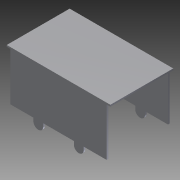
# Autodesk Inventor part: M20_ang_t_shorud1230TX-switch
Saved by Autodesk Inventor 2011 SP1 (Build 150282100, 282)
## iProperties
Created: 2013-12-24
Part Number: M20_ang_t_shorud1230TX-switch
Catalog Web Link: www.cadenas.de
Description: Angle Mount Miniature Rockers- Switch - Shroud-Series M - Miniature Toggle
Vendor: NKKSWITCHES
Document SubType Name: Modeling
Designer: PARTuser1
Manufacturer: NKKSWITCHES
Density: 1 g/cm^3
Category: PARTsolutions
Company: NKKSWITCHES
Title: M20_ang_t_shorud1230TX-switch
Author: Cadenas PARTsolutions
Comments: Series M - Miniature Toggle
PSOL_IDENT_0: {$CADENAS_DATA\23d-libs\nkkswitches\toggle\m\parts\m_ang_t_shroud.prj},260 {VTYP=3D},{NB=M20_ang_t_s
PSOL_IDENT_1: horud1230TX-switch},{LINA=M20_ang_t_shorud1230TX-switch},{NN=Angle Mount Miniature Rockers- Switch -
PSOL_IDENT_2: Shroud},{DATE=28.05.2007 07:44:41},{GEOMDATE=28.05.2007 00:00:00},{VERSION=},{LINEID=10},{LINESUBID
PSOL_IDENT_3: =-1},{WBVAR=PLS,CRCTS,FRM,TRMNLS}  {NB=M20_ang_t_shorud1230TX-switch},{LINA=M20_ang_t_shorud1230TX-s
PSOL_IDENT_4: witch},{KT=DUMMY},{PN=M20_ang_t_shorud1230TX},{SRS=M20},{PLS=1},{CRCTSALG='2','2 - ON/NONE/ON','3','
PSOL_IDENT_5: 3 - ON/OFF/ON','5','5 - ON/NONE/(ON)','8','8 - (ON)/OFF/(ON)','9','9 - ON/OFF/(ON)','4', '4 - ON/ON/
PSOL_IDENT_6: ON','6','6 - (ON)/ON/(ON)','7','7 - ON/ON/(ON)'},{CRCTS=2},{FRMALG='TX', 'TX - Narrow Frame for Smal
PSOL_IDENT_7: l Actuator', 'TZ'  , 'TZ - Wide Frame for Large Actuator'},{FRM=TX},{TRMNLSALG='30', '30 - .150\" (3
PSOL_IDENT_8: .81mm) Right Angle PC (1-3 Pole)', '32'  , '32 -  Right Angle PCB (1 Pole & 0.4VA Rating Only', '40'
PSOL_IDENT_9: , '40 - .150\" (3.81mm) Vertical PC (1-4 Pole)', '45'  , '45 - .100\" (2.54mm) Vertical PC (1-4 Po
PSOL_IDENT_10: le)'},{TRMNLS=30},{WIDTH=0.512},{HEIGHT=0.3877},{LENGTH=0.311},{A=0.15},{TRMNLNOH=1},{TRMNLOV=3},{LT
PSOL_IDENT_11: RMNL=0.031},{POS=0},{POS2=0.185},{POS3=0},{D=0},{HOLES=0.185},{WH=0.00000},{D1=0.00000},{D2=0.00000}
CNS_NN: Angle Mount Miniature Rockers- Switch - Shroud
CNS_NT: Series M - Miniature Toggle
CNS_NB: M20_ang_t_shorud1230TX-switch
CNS_NBSYN: $PN.-switch
CNS_LINA: M20_ang_t_shorud1230TX-switch
CNS_PN: M20_ang_t_shorud1230TX
CNS_SRS: M20
CNS_PLS: 1 - SPST/SPDT
CNS_CRCTSALG: '2','2 - ON/NONE/ON','3','3 - ON/OFF/ON','5','5 - ON/NONE/(ON)','8','8 - (ON)/OFF/(ON)','9','9 - ON/OFF/(ON)','4', '4 - ON/ON/ON','6','6 - (ON)/ON/(ON)','7','7 - ON/ON/(ON)'
CNS_CRCTS: 2 - ON/NONE/ON
CNS_FRMALG: 'TX', 'TX - Narrow Frame for Small Actuator', 'TZ'  , 'TZ - Wide Frame for Large Actuator'
CNS_FRM: TX - Narrow Frame for Small Actuator
CNS_TRMNLSALG: '30', '30 - .150" (3.81mm) Right Angle PC (1-3 Pole)', '32'  , '32 -  Right Angle PCB (1 Pole & 0.4VA Rating Only', '40'  , '40 - .150" (3.81mm) Vertical PC (1-4 Pole)', '45'  , '45 - .100" (2.54mm) Vertical PC (1-4 Pole)'
CNS_TRMNLS: 30 - .150" (3.81mm) Right Angle PC (1-3 Pole)
CNS_WIDTH: 0.512
CNS_HEIGHT: 0.388
CNS_LENGTH: 0.311
CNS_A: 0.150
CNS_TRMNLNOH: 1.000
CNS_TRMNLOV: 3.000
CNS_LTRMNL: 0.031
CNS_POS: 0.000
CNS_POS2: 0.185
CNS_POS3: 0.000
CNS_D: 0.000
CNS_HOLES: 0.185
CNS_WH: 0.00000
CNS_D1: 0.00000
CNS_D2: 0.00000
SUPPLIER: NKKSWITCHES
ARTICLENO: M20_ang_t_shorud1230TX-switch
BOMINFO: M20_ang_t_shorud1230TX-switch
CREATOR: CADENAS GmbH
Autodesk Inventor part; units mm, degrees
sketch "Sketch_1" plane through (0, 0, 0) normal (0, 1, 0) x (-1, 0, 0)
  line L0 (6.5024, 3.9497) -> (-6.5024, 3.9497)
  line L1 (-6.5024, 3.9497) -> (-6.5024, -3.9497)
  line L2 (-6.5024, -3.9497) -> (6.5024, -3.9497)
  line L3 (6.5024, -3.9497) -> (6.5024, 3.9497)
  constraints: 8 end point
extrude "Extrusion1" add sketch "Sketch_1" along normal blind 0.2032
sketch "Sketch_2" plane through (0, 0, -3.9497) normal (0, 0, 1) x (1, 0, 0)
  line L0 (-6.0389, -6.018) -> (-3.1581, -6.018)
  line L1 (-3.1581, -6.018) -> (-3.1581, -6.4159)
  arc A0 (-3.1581, -6.4159) -> (-1.9219, -6.4159) centre (-2.54, -6.4159) ccw
  line L2 (-1.9219, -6.4159) -> (-1.9219, -6.018)
  line L3 (-1.9219, -6.018) -> (1.9219, -6.018)
  line L4 (1.9219, -6.018) -> (1.9219, -6.4159)
  arc A1 (1.9219, -6.4159) -> (3.1581, -6.4159) centre (2.54, -6.4159) ccw
  line L5 (3.1581, -6.4159) -> (3.1581, -6.018)
  line L6 (3.1581, -6.018) -> (6.0389, -6.018)
  line L7 (6.0389, -6.018) -> (6.0389, 0)
  line L8 (6.0389, 0) -> (-6.0389, 0)
  line L9 (-6.0389, 0) -> (-6.0389, -6.018)
  constraints: 20 end point, 4 point on circle, 2 centre point
extrude "Extrusion2" add sketch "Sketch_2" along normal blind 0.2032
sketch "Sketch_3" plane through (0, 0, 3.9497) normal (0, 0, 1) x (1, 0, 0)
  line L0 (-6.0389, -6.018) -> (-3.1581, -6.018)
  line L1 (-3.1581, -6.018) -> (-3.1581, -6.4159)
  arc A0 (-3.1581, -6.4159) -> (-1.9219, -6.4159) centre (-2.54, -6.4159) ccw
  line L2 (-1.9219, -6.4159) -> (-1.9219, -6.018)
  line L3 (-1.9219, -6.018) -> (1.9219, -6.018)
  line L4 (1.9219, -6.018) -> (1.9219, -6.4159)
  arc A1 (1.9219, -6.4159) -> (3.1581, -6.4159) centre (2.54, -6.4159) ccw
  line L5 (3.1581, -6.4159) -> (3.1581, -6.018)
  line L6 (3.1581, -6.018) -> (6.0389, -6.018)
  line L7 (6.0389, -6.018) -> (6.0389, 0)
  line L8 (6.0389, 0) -> (-6.0389, 0)
  line L9 (-6.0389, 0) -> (-6.0389, -6.018)
  constraints: 20 end point, 4 point on circle, 2 centre point
extrude "Extrusion3" add sketch "Sketch_3" against normal blind 0.2032
ref_plane "shroud_to_body_XY" through (0, 0, 0) normal (0, 1, 0) x (1, 0, 0)
ref_plane "shroud_to_body_YZ" through (0, 0, 0) normal (1, 0, 0) x (0, 0, -1)
ref_plane "shroud_to_body_ZX" through (0, 0, 0) normal (0, 0, -1) x (0, 1, 0)
body "Solid1"
